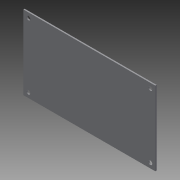
# Autodesk Inventor part: Microzed01
Saved by Autodesk Inventor 2013 (Build 170138000, 138)
## iProperties
Created: 2014-04-13
Part Number: Microzed01
Material: PCB(1)
Document SubType Name: Modeling
Designer: spichelh
Density: 1 g/cm^3
Author: spichelh
Autodesk Inventor part; units mm, degrees
ref_plane "YZ Plane" through (0, 0, 0) normal (1, 0, 0) x (0, 1, 0)
ref_plane "XZ Plane" through (0, 0, 0) normal (0, 1, 0) x (-1, 0, 0)
ref_plane "XY Plane" through (0, 0, 0) normal (0, 0, 1) x (1, 0, 0)
sketch "Sketch1" plane through (0, 0, 0) normal (0, 0, 1) x (1, 0, 0)
  line L0 (-50.8, -28.575) -> (50.8, -28.575)
  line L1 (50.8, -28.575) -> (50.8, 28.575)
  line L2 (50.8, 28.575) -> (-50.8, 28.575)
  line L3 (-50.8, 28.575) -> (-50.8, -28.575)
  line L4 (-50.8, -28.575) -> (50.8, 28.575) construction
  line L5 (50.8, -28.575) -> (-50.8, 28.575) construction
  circle A0 centre (-46.99, 24.765) radius 1.5
  line L6 (-50.8, 0) -> (50.8, 0) construction
  line L7 (0, 28.575) -> (0, -28.575) construction
  circle A1 centre (-46.99, -24.765) radius 1.5
  circle A2 centre (46.99, 24.765) radius 1.5
  circle A3 centre (46.99, -24.765) radius 1.5
  point P0 (0, 0)
  dimension "d2" = 101.6
  dimension "d4" = 57.15
  dimension "d5" = 49.53
  dimension "d6" = 3
  dimension "d7" = 93.98
  constraints: 16 end point, 6 midpoint, 4 centre point, 3 symmetric about line, 2 parallel, 1 horizontal, 1 perpendicular, 3 other
  measures "d2" distance of L1.end L2.end
  measures "d4" distance of L0.end L1.end
  measures "d5" distance of A1.centre A0.centre
  measures "d6" diameter of A1
  measures "d7" distance of A2.centre A0.centre
extrude "Extrusion1" add sketch "Sketch1" along normal blind 1
body "Solid1"
